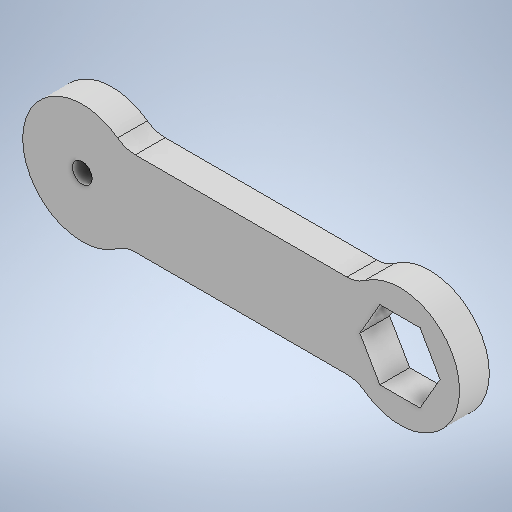
# Autodesk Inventor part: 2P.03.01.16.ZW.FlapCrank
Saved by Autodesk Inventor 2025.2 (Build 292293000, 293)
## iProperties
Created: 2025-01-14
Part Number: 2P.03.01.16.ZW.FlapCrank
Material: Generic
Document SubType Name: Modeling
Designer: Imist
Density: 1 g/cm^3
Appearance: Default
Author: Imist
Autodesk Inventor part; units mm, degrees
ref_plane "YZ Plane" through (0, 0, 0) normal (1, 0, 0) x (0, 1, 0)
ref_plane "XZ Plane" through (0, 0, 0) normal (0, 1, 0) x (-1, 0, 0)
ref_plane "XY Plane" through (0, 0, 0) normal (0, 0, 1) x (1, 0, 0)
sketch "Sketch1" plane through (0, 0, 0) normal (0, 0, 1) x (1, 0, 0)
  circle A0 centre (15.9778, 0.0222) radius 3.5
  arc A1 (-16.0222, 6.0222) -> (-16.0222, -5.9778) centre (-16.0222, 0.0222) ccw
  arc A2 (15.9778, -5.9778) -> (15.9778, 6.0222) centre (15.9778, 0.0222) ccw
  arc A3 (-16.0222, -5.9778) -> (-12.4604, -4.8063) centre (-16.0222, 0.0222) ccw
  line L0 (-16.0222, 0.0222) -> (-11.7795, -4.2205) construction
  line L1 (-16.0222, 0.0222) -> (-16.0222, -5.9778) construction
  arc A4 (-12.4604, 4.8506) -> (-16.0222, 6.0222) centre (-16.0222, 0.0222) ccw
  line L2 (-16.0222, 0.0222) -> (-11.7795, 4.2648) construction
  line L3 (-16.0222, 0.0222) -> (-16.0222, 6.0222) construction
  arc A5 (15.9778, 6.0222) -> (12.4161, 4.8506) centre (15.9778, 0.0222) ccw
  line L4 (15.9778, 0.0222) -> (11.7352, 4.2648) construction
  line L5 (15.9778, 0.0222) -> (15.9778, 6.0222) construction
  arc A6 (12.4161, -4.8063) -> (15.9778, -5.9778) centre (15.9778, 0.0222) ccw
  line L6 (15.9778, 0.0222) -> (11.7352, -4.2205) construction
  line L7 (15.9778, 0.0222) -> (15.9778, -5.9778) construction
  line L8 (-10.6795, 4.2648) -> (10.6352, 4.2648)
  line L9 (-10.6795, -4.2205) -> (10.6352, -4.2205)
  arc A7 (-12.4604, 4.8506) -> (-10.6795, 4.2648) centre (-10.6795, 7.2648) ccw
  arc A8 (-10.6795, -4.2205) -> (-12.4604, -4.8063) centre (-10.6795, -7.2205) ccw
  arc A9 (10.6352, 4.2648) -> (12.4161, 4.8506) centre (10.6352, 7.2648) ccw
  arc A10 (12.4161, -4.8063) -> (10.6352, -4.2205) centre (10.6352, -7.2205) ccw
  line L10 (11.9364, 0.0222) -> (13.9571, 3.5222)
  line L11 (13.9571, 3.5222) -> (17.9986, 3.5222)
  line L12 (17.9986, 3.5222) -> (20.0193, 0.0222)
  line L13 (20.0193, 0.0222) -> (17.9986, -3.4778)
  line L14 (17.9986, -3.4778) -> (13.9571, -3.4778)
  line L15 (13.9571, -3.4778) -> (11.9364, 0.0222)
  circle A11 centre (-16.0222, 0.0222) radius 1
  point P0 (0, 0)
  dimension "d1" = 7
  dimension "d2" = 32
  dimension "d3" = 6
  dimension "d4" = 6
  dimension "d5" = 45
  dimension "d6" = 45
  dimension "d7" = 45
  dimension "d8" = 45
  dimension "d9" = 3
  dimension "d14" = 2
  constraints: 32 end point, 24 point on circle, 12 centre point, 9 tangent, 8 coincident, 4 point on line, 3 equal radius, 1 horizontal, 13 other
  measures "d1" diameter of A0
  measures "d2" distance of L1.end L7.end
  measures "d3" radius of A1
  measures "d4" radius of A2
  measures "d5" angle of L1 L0
  measures "d6" angle of L2 L3
  measures "d7" angle of L5 L4
  measures "d8" angle of L6 L7
  measures "d9" radius of A7
  measures "d14" diameter of A11
extrude "Extrusion2" add sketch "Sketch1" along normal blind 3
body "Solid2"
